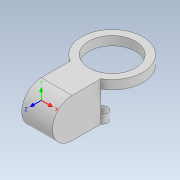
# Autodesk Inventor part: hip_back_left
Saved by Autodesk Inventor 2020 (Build 240168000, 168)
## iProperties
Created: 2021-01-12
Part Number: hip_back_left
Material: Generic
Document SubType Name: Modeling
Designer: DELL
Density: 1 g/cm^3
Appearance: Default
Author: DELL
Autodesk Inventor part; units mm, degrees
ref_plane "YZ Plane" through (0, 0, 0) normal (1, 0, 0) x (0, 1, 0)
ref_plane "XY Plane" through (0, 0, 0) normal (0, 0, 1) x (1, 0, 0)
ref_plane "UCS1: YZ Plane" through (0, 0, 0) normal (1, 0, 0) x (0, 1, 0)
sketch "Sketch2" plane through (0, 0, 0) normal (0, 1, 0) x (-1, 0, 0)
  circle A0 centre (-20.75, -75) radius 36 construction
  line L0 (-20.75, -75) -> (-56.75, -75) construction
  line L1 (-20.75, -75) -> (8.9441, -54.6466) construction
  circle A1 centre (-20.75, -75) radius 41.5
  circle A2 centre (-20.75, -75) radius 28
  arc A3 (-6.75, -50.7513) -> (0, -39.0599) centre (-3.375, -44.9056) ccw
  arc A4 (-41.5, -39.0599) -> (-31.4929, -46.1619) centre (-38.125, -44.9056) ccw
  line L2 (-20.75, -75) -> (-3.375, -44.9056) construction
  circle A5 centre (-20.75, -75) radius 31.5
  line L3 (0, -39.0599) -> (0, 0)
  line L4 (-41.5, -39.0599) -> (-41.5, 0)
  line L5 (0, 0) -> (-41.5, 0)
  line L6 (-20.75, 0) -> (-20.75, -75) construction
  point P0 (20.2329, -68.469)
  point P1 (18.0842, -60.366)
  point P2 (-31.3991, -44.3363)
  point P3 (-34.75, -50.7513)
  dimension "d1" = 72
  dimension "d5" = 83
  dimension "d6" = 56
  dimension "d7" = 63
  dimension "d11" = 41.5
  dimension "d31" = 75
  constraints: 15 end point, 11 point on circle, 6 centre point, 4 coincident, 4 tangent, 3 vertical, 1 horizontal, 1 midpoint, 1 point on line
  measures "d1" diameter of A0
  measures "d5" diameter of A1
  measures "d6" diameter of A2
  measures "d7" diameter of A5
  measures "d11" distance of L3.end L4.end
  measures "d31" distance from line of L5 A1.centre
ref_plane "Work Plane1" through (0, -14.5, 0) normal (0, 1, 0) x (-1, 0, 0)
ref_plane "Work Plane2" through (0, 14.5, 0) normal (0, 1, 0) x (-1, 0, 0)
extrude "Extrusion1" add sketch "Sketch2" along normal blind 12 from surface at 14.5 contours A1 A4 A5 A3 | A3 A5 A4 A1
extrude "Extrusion2" add sketch "Sketch2" against normal blind 12 from surface at -14.5 contours A3 A5 A4 A1 | A3 A2 A4 A5 picked at (-36.682, -40.4948) picked at (-30.8117, -46.5413)
extrude "Extrusion3" add sketch "Sketch2" along normal mid plane 53 contours A1 L4 L5 L3
sketch "Sketch3" plane through (0, 0, 0) normal (1, 0, 0) x (0, 1, 0)
  line L0 (-26.5, 0) -> (26.5, 0) projected
  circle A0 centre (0, 0) radius 26.5
  constraints: 1 coincident, 1 horizontal alignment, 2 other
extrude "Extrusion4" add sketch "Sketch3" along normal up to surface (41.5 mm away)
body "Solid1"
